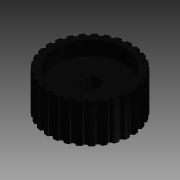
# Autodesk Inventor part: Llave hornillo
Saved by Autodesk Inventor 2014 (Build 180170000, 170)
## iProperties
Created: 2017-05-23
Part Number: Llave hornillo
Material: Generic
Document SubType Name: Modeling
Designer: resaj
Density: 1 g/cm^3
Appearance: Smooth - Black
Author: resaj
Autodesk Inventor part; units mm, degrees
ref_plane "YZ Plane" through (0, 0, 0) normal (1, 0, 0) x (0, 1, 0)
ref_plane "XZ Plane" through (0, 0, 0) normal (0, 1, 0) x (-1, 0, 0)
ref_plane "XY Plane" through (0, 0, 0) normal (0, 0, 1) x (1, 0, 0)
sketch "Sketch1" plane through (0, 0, 0) normal (0, 1, 0) x (-1, 0, 0)
  circle A0 centre (0, 0) radius 18.5
  dimension "d0" = 37
  constraints: 1 centre point, 1 coincident
  measures "d0" diameter of A0
extrude "Extrusion1" add sketch "Sketch1" along normal blind 17
sketch "Sketch2" plane through (0, 17, 0) normal (0, 1, 0) x (1, 0, 0)
  circle A0 centre (0, 0) radius 18.5 projected
  circle A1 centre (18.5, 0) radius 1
  line L0 (0, 0) -> (18.5, 0) construction
  dimension "d3" = 2
  constraints: 2 end point, 1 centre point, 1 horizontal, 1 horizontal alignment, 1 other
  measures "d3" diameter of A1
extrude "Extrusion2" cut sketch "Sketch2" against normal through all contours A0 A1 | A0 A1 picked at (18.1866, 0.2274) picked at (18.7982, 0.2581)
pattern_circular "Circular Pattern1" count 29 over 360 about axis through (0, 0, 0) along (0, 1, 0) of "Extrusion2"
sketch "Sketch3" plane through (0, 0, 0) normal (0, -1, 0) x (1, 0, 0)
  arc A0 (17.8262, 4.9474) -> (17.1854, 6.8494) centre (0, 0) ccw projected
hole "Hole1" at (0, 0, 0) direction (0, 1, 0) diameter 3.5 end through all countersink diameter 9.5 countersink angle 90
sketch "Sketch4" plane through (0, 0, 0) normal (0, -1, 0) x (1, 0, 0)
  circle A0 centre (0, 0) radius 4.75 projected
  arc A1 (-18.4728, 1.0035) -> (-18.4728, -1.0035) centre (0, 0) ccw projected
  arc A2 (18.473, 0.9996) -> (18.256, 2.9949) centre (0, 0) ccw projected
  line L0 (-9.6, 0.7) -> (-5.75, 0.7)
  line L1 (-5.75, 0.7) -> (-5.75, -0.7)
  line L2 (-5.75, -0.7) -> (-9.6, -0.7)
  line L3 (-9.6, -0.7) -> (-9.6, 0.7)
  line L4 (-18.5, 0) -> (0, 0) construction
  line L5 (-7.675, 0.7) -> (-7.675, 0) construction
  line L6 (-7.675, 0) -> (-7.675, -0.7) construction
  circle A3 centre (0, 0) radius 11.4692 construction
  line L7 (-0.2594, 7.791) -> (2.8062, 7.791) construction
  line L8 (2.8062, 7.791) -> (2.8062, 10.4034) construction
  line L9 (2.8062, 10.4034) -> (0.8969, 11.8689) construction
  line L10 (0.8969, 11.8689) -> (0.2634, 13.3204) construction
  line L11 (0.2634, 13.3204) -> (-0.0505, 15.6348) construction
  spline S0 degree 4 poles (-0.2594, 7.791) (2.8062, 7.791) (2.8062, 10.4034) (0.8969, 11.8689) (0.2634, 13.3204) (-0.0505, 15.6348) knots 1 1 1 1 1 2 3 3 3 3 3
  line L12 (-0.2594, 7.791) -> (-3.3031, 7.791) construction
  line L13 (-3.3031, 7.791) -> (-4.0256, 9.1624) construction
  line L14 (-4.0256, 9.1624) -> (-3.2524, 11.7471) construction
  spline S1 degree 3 poles (-0.2594, 7.791) (-3.3031, 7.791) (-4.0256, 9.1624) (-3.2524, 11.7471) knots 1 1 1 1 2 2 2 2
  line L15 (-3.2524, 11.7471) -> (-2.5295, 10.0909) construction
  line L16 (-2.5295, 10.0909) -> (-2.3206, 10.0909) construction
  line L17 (-2.3206, 10.0909) -> (-2.3206, 12.6773) construction
  line L18 (-2.3206, 12.6773) -> (-0.0505, 15.6348) construction
  spline S2 degree 4 poles (-3.2524, 11.7471) (-2.5295, 10.0909) (-2.3206, 10.0909) (-2.3206, 12.6773) (-0.0505, 15.6348) knots 1 1 1 1 1 2 2 2 2 2
  line L19 (5.6325, 5.7441) -> (6.9202, 4.4564) construction
  line L20 (6.9202, 4.4564) -> (8.0174, 5.5537) construction
  line L21 (8.0174, 5.5537) -> (7.8311, 6.9712) construction
  line L22 (7.8311, 6.9712) -> (8.1746, 7.8469) construction
  line L23 (8.1746, 7.8469) -> (9.0149, 8.9509) construction
  spline S3 degree 4 poles (5.6325, 5.7441) (6.9202, 4.4564) (8.0174, 5.5537) (7.8311, 6.9712) (8.1746, 7.8469) (9.0149, 8.9509) knots 1 1 1 1 1 2 3 3 3 3 3
  line L24 (5.6325, 5.7441) -> (4.354, 7.0226) construction
  line L25 (4.354, 7.0226) -> (4.6267, 7.9019) construction
  line L26 (4.6267, 7.9019) -> (6.0371, 8.6628) construction
  spline S4 degree 3 poles (5.6325, 5.7441) (4.354, 7.0226) (4.6267, 7.9019) (6.0371, 8.6628) knots 1 1 1 1 2 2 2 2
  line L27 (6.0371, 8.6628) -> (5.6451, 7.6636) construction
  line L28 (5.6451, 7.6636) -> (5.7328, 7.5758) construction
  line L29 (5.7328, 7.5758) -> (6.8191, 8.6622) construction
  line L30 (6.8191, 8.6622) -> (9.0149, 8.9509) construction
  spline S5 degree 4 poles (6.0371, 8.6628) (5.6451, 7.6636) (5.7328, 7.5758) (6.8191, 8.6622) (9.0149, 8.9509) knots 1 1 1 1 1 2 2 2 2 2
  arc A4 (18.256, -2.9949) -> (18.473, -0.9996) centre (0, 0) ccw projected
  line L31 (0, 0) -> (13.0815, 13.0815) construction
  line L32 (0, 0) -> (18.5, 0) construction
  spline S6 degree 2 poles (-10.161, -5.2239) (-10.0622, -5.4091) (-10.0419, -5.8018) (-10.129, -5.9928) knots 0 0 0 1 2 2 2
  spline S7 degree 2 poles (-10.129, -5.9928) (-10.2133, -6.1847) (-10.5824, -6.5424) (-10.8658, -6.6935) knots 0 0 0 1 2 2 2
  spline S8 degree 2 poles (-10.8658, -6.6935) (-11.1473, -6.8436) (-11.63, -6.9445) (-11.8463, -6.9106) knots 0 0 0 1 2 2 2
  spline S9 degree 2 poles (-11.8463, -6.9106) (-12.0571, -6.8783) (-12.3817, -6.6502) (-12.4843, -6.4576) knots 0 0 0 1 2 2 2
  spline S10 degree 2 poles (-12.4843, -6.4576) (-12.5356, -6.3614) (-12.592, -6.1768) (-12.6053, -6.0906) knots 0 0 0 1 2 2 2
  spline S11 degree 2 poles (-12.6053, -6.0906) (-12.6136, -6.0181) (-12.6161, -5.8515) (-12.6091, -5.7684) knots 0 0 0 1 2 2 2
  line L33 (-12.6091, -5.7684) -> (-12.2495, -5.5767)
  line L34 (-12.2495, -5.5767) -> (-12.2388, -5.5967)
  spline S12 degree 2 poles (-12.2388, -5.5967) (-12.2567, -5.6506) (-12.3033, -5.8083) (-12.3116, -5.9107) knots 0 0 0 1 2 2 2
  spline S13 degree 2 poles (-12.3116, -5.9107) (-12.3201, -6.0086) (-12.2891, -6.2113) (-12.229, -6.3239) knots 0 0 0 1 2 2 2
  spline S14 degree 2 poles (-12.229, -6.3239) (-12.1642, -6.4456) (-11.9309, -6.5988) (-11.7747, -6.6205) knots 0 0 0 1 2 2 2
  spline S15 degree 2 poles (-11.7747, -6.6205) (-11.6167, -6.6412) (-11.2223, -6.5453) (-11.0062, -6.4301) knots 0 0 0 1 2 2 2
  spline S16 degree 2 poles (-11.0062, -6.4301) (-10.7755, -6.3071) (-10.4934, -6.0355) (-10.4226, -5.8928) knots 0 0 0 1 2 2 2
  spline S17 degree 2 poles (-10.4226, -5.8928) (-10.3544, -5.7538) (-10.356, -5.4794) (-10.4199, -5.3595) knots 0 0 0 1 2 2 2
  spline S18 degree 2 poles (-10.4199, -5.3595) (-10.479, -5.2487) (-10.6413, -5.0973) (-10.7273, -5.0499) knots 0 0 0 1 2 2 2
  spline S19 degree 2 poles (-10.7273, -5.0499) (-10.8122, -5.0042) (-10.9645, -4.9548) (-11.0145, -4.9441) knots 0 0 0 1 2 2 2
  line L35 (-11.0145, -4.9441) -> (-11.0252, -4.9241)
  line L36 (-11.0252, -4.9241) -> (-10.6692, -4.7343)
  spline S20 degree 2 poles (-10.6692, -4.7343) (-10.6018, -4.7777) (-10.4781, -4.8564) (-10.4075, -4.919) knots 0 0 0 1 2 2 2
  spline S21 degree 2 poles (-10.4075, -4.919) (-10.3302, -4.9852) (-10.222, -5.1094) (-10.161, -5.2239) knots 0 0 0 1 2 2 2
  line L37 (-10.6086, -4.402) -> (-13.0032, -5.2488)
  line L38 (-13.0032, -5.2488) -> (-13.4534, -3.9757)
  line L39 (-13.4534, -3.9757) -> (-13.1701, -3.8755)
  line L40 (-13.1701, -3.8755) -> (-12.8153, -4.8788)
  line L41 (-12.8153, -4.8788) -> (-12.1594, -4.6469)
  line L42 (-12.1594, -4.6469) -> (-12.4901, -3.7115)
  line L43 (-12.4901, -3.7115) -> (-12.2068, -3.6113)
  line L44 (-12.2068, -3.6113) -> (-11.8761, -4.5467)
  line L45 (-11.8761, -4.5467) -> (-10.9873, -4.2324)
  line L46 (-10.9873, -4.2324) -> (-11.342, -3.2291)
  line L47 (-11.342, -3.2291) -> (-11.0587, -3.1289)
  line L48 (-11.0587, -3.1289) -> (-10.6086, -4.402)
  line L49 (-11.4486, -1.187) -> (-11.3791, -1.553)
  line L50 (-11.3791, -1.553) -> (-12.2447, -2.4128)
  line L51 (-12.2447, -2.4128) -> (-12.1837, -2.7343)
  line L52 (-12.1837, -2.7343) -> (-11.1908, -2.546)
  line L53 (-11.1908, -2.546) -> (-11.1374, -2.8271)
  line L54 (-11.1374, -2.8271) -> (-13.6329, -3.3005)
  line L55 (-13.6329, -3.3005) -> (-13.7365, -2.7544)
  spline S22 degree 2 poles (-13.7365, -2.7544) (-13.771, -2.5724) (-13.7713, -2.3169) (-13.7075, -2.1895) knots 0 0 0 1 2 2 2
  spline S23 degree 2 poles (-13.7075, -2.1895) (-13.6437, -2.0622) (-13.4033, -1.8825) (-13.2071, -1.8453) knots 0 0 0 1 2 2 2
  spline S24 degree 2 poles (-13.2071, -1.8453) (-12.9341, -1.7935) (-12.5192, -1.9599) (-12.3914, -2.1473) knots 0 0 0 1 2 2 2
  line L56 (-12.3914, -2.1473) -> (-11.4486, -1.187)
  spline S25 degree 2 poles (-13.1252, -2.1336) (-13.2344, -2.1543) (-13.39, -2.2508) (-13.4316, -2.33) knots 0 0 0 1 2 2 2
  spline S26 degree 2 poles (-13.4316, -2.33) (-13.4666, -2.3994) (-13.4747, -2.5665) (-13.452, -2.6858) knots 0 0 0 1 2 2 2
  line L57 (-13.452, -2.6858) -> (-13.3991, -2.9649)
  line L58 (-13.3991, -2.9649) -> (-12.4608, -2.7869)
  line L59 (-12.4608, -2.7869) -> (-12.5079, -2.5381)
  spline S27 degree 2 poles (-12.5079, -2.5381) (-12.531, -2.4168) (-12.6183, -2.2323) (-12.7103, -2.1785) knots 0 0 0 1 2 2 2
  spline S28 degree 2 poles (-12.7103, -2.1785) (-12.7905, -2.1308) (-12.9958, -2.109) (-13.1252, -2.1336) knots 0 0 0 1 2 2 2
  line L60 (-11.4914, 0.6533) -> (-11.4812, 0.2809)
  line L61 (-11.4812, 0.2809) -> (-12.4728, -0.4299)
  line L62 (-12.4728, -0.4299) -> (-12.4638, -0.7571)
  line L63 (-12.4638, -0.7571) -> (-11.4535, -0.7294)
  line L64 (-11.4535, -0.7294) -> (-11.4457, -1.0154)
  line L65 (-11.4457, -1.0154) -> (-13.9848, -1.0849)
  line L66 (-13.9848, -1.0849) -> (-14, -0.5294)
  spline S29 degree 2 poles (-14, -0.5294) (-14.005, -0.3442) (-13.9646, -0.0919) (-13.8812, 0.0237) knots 0 0 0 1 2 2 2
  spline S30 degree 2 poles (-13.8812, 0.0237) (-13.7979, 0.1392) (-13.532, 0.2783) (-13.3324, 0.2837) knots 0 0 0 1 2 2 2
  spline S31 degree 2 poles (-13.3324, 0.2837) (-13.0546, 0.2913) (-12.6715, 0.0609) (-12.5753, -0.1444) knots 0 0 0 1 2 2 2
  line L67 (-12.5753, -0.1444) -> (-11.4914, 0.6533)
  spline S32 degree 2 poles (-13.2975, -0.0139) (-13.4086, -0.0169) (-13.5776, -0.0874) (-13.6312, -0.1589) knots 0 0 0 1 2 2 2
  spline S33 degree 2 poles (-13.6312, -0.1589) (-13.6769, -0.2219) (-13.7115, -0.3856) (-13.7082, -0.507) knots 0 0 0 1 2 2 2
  line L68 (-13.7082, -0.507) -> (-13.7004, -0.7909)
  line L69 (-13.7004, -0.7909) -> (-12.7457, -0.7648)
  line L70 (-12.7457, -0.7648) -> (-12.7526, -0.5117)
  spline S34 degree 2 poles (-12.7526, -0.5117) (-12.756, -0.3882) (-12.8128, -0.1921) (-12.895, -0.1244) knots 0 0 0 1 2 2 2
  spline S35 degree 2 poles (-12.895, -0.1244) (-12.9666, -0.0645) (-13.1658, -0.0103) (-13.2975, -0.0139) knots 0 0 0 1 2 2 2
  line L71 (-11.4907, 0.5916) -> (-13.9137, 1.6445)
  line L72 (-13.9137, 1.6445) -> (-13.8673, 1.9955)
  line L73 (-13.8673, 1.9955) -> (-11.254, 2.3833)
  line L74 (-11.254, 2.3833) -> (-11.2936, 2.0833)
  line L75 (-11.2936, 2.0833) -> (-12.0233, 1.9824)
  line L76 (-12.0233, 1.9824) -> (-12.1313, 1.1641)
  line L77 (-12.1313, 1.1641) -> (-11.4529, 0.8773)
  line L78 (-11.4529, 0.8773) -> (-11.4907, 0.5916)
  line L79 (-12.3192, 1.9426) -> (-13.5525, 1.7692)
  line L80 (-13.5525, 1.7692) -> (-12.4065, 1.2814)
  line L81 (-12.4065, 1.2814) -> (-12.3192, 1.9426)
  spline S36 degree 2 poles (-11.9106, 4.605) (-11.578, 4.5031) (-11.1127, 4.1108) (-11.0222, 3.8721) knots 0 0 0 1 2 2 2
  spline S37 degree 2 poles (-11.0222, 3.8721) (-10.9537, 3.681) (-10.9739, 3.3341) (-11.0511, 3.0822) knots 0 0 0 1 2 2 2
  line L82 (-11.0511, 3.0822) -> (-11.1965, 2.6079)
  line L83 (-11.1965, 2.6079) -> (-13.625, 3.3522)
  line L84 (-13.625, 3.3522) -> (-13.4808, 3.8225)
  spline S38 degree 2 poles (-13.4808, 3.8225) (-13.3922, 4.1118) (-13.1885, 4.4111) (-13.0618, 4.5014) knots 0 0 0 1 2 2 2
  spline S39 degree 2 poles (-13.0618, 4.5014) (-12.8454, 4.6526) (-12.2648, 4.7136) (-11.9106, 4.605) knots 0 0 0 1 2 2 2
  spline S40 degree 2 poles (-12.002, 4.3209) (-12.2814, 4.4065) (-12.7252, 4.3703) (-12.8851, 4.2492) knots 0 0 0 1 2 2 2
  spline S41 degree 2 poles (-12.8851, 4.2492) (-12.9956, 4.1625) (-13.1405, 3.9357) (-13.1978, 3.7487) knots 0 0 0 1 2 2 2
  line L85 (-13.1978, 3.7487) -> (-13.2617, 3.5401)
  line L86 (-13.2617, 3.5401) -> (-11.3921, 2.9671)
  line L87 (-11.3921, 2.9671) -> (-11.3282, 3.1757)
  spline S42 degree 2 poles (-11.3282, 3.1757) (-11.2721, 3.3588) (-11.2565, 3.6554) (-11.3146, 3.7959) knots 0 0 0 1 2 2 2
  spline S43 degree 2 poles (-11.3146, 3.7959) (-11.3847, 3.9746) (-11.7186, 4.234) (-12.002, 4.3209) knots 0 0 0 1 2 2 2
  spline S44 degree 2 poles (-11.8745, 6.9059) (-11.6679, 6.9383) (-11.1666, 6.8327) (-10.8848, 6.6874) knots 0 0 0 1 2 2 2
  spline S45 degree 2 poles (-10.8848, 6.6874) (-10.6104, 6.5459) (-10.2272, 6.1978) (-10.1347, 6.0089) knots 0 0 0 1 2 2 2
  spline S46 degree 2 poles (-10.1347, 6.0089) (-10.0377, 5.8107) (-10.049, 5.4205) (-10.1461, 5.232) knots 0 0 0 1 2 2 2
  spline S47 degree 2 poles (-10.1461, 5.232) (-10.247, 5.0363) (-10.5629, 4.8054) (-10.7732, 4.7703) knots 0 0 0 1 2 2 2
  spline S48 degree 2 poles (-10.7732, 4.7703) (-10.9798, 4.7379) (-11.4821, 4.8463) (-11.7601, 4.9896) knots 0 0 0 1 2 2 2
  spline S49 degree 2 poles (-11.7601, 4.9896) (-12.0437, 5.1358) (-12.4132, 5.4792) (-12.5122, 5.6691) knots 0 0 0 1 2 2 2
  spline S50 degree 2 poles (-12.5122, 5.6691) (-12.6046, 5.8581) (-12.5989, 6.2511) (-12.4989, 6.445) knots 0 0 0 1 2 2 2
  spline S51 degree 2 poles (-12.4989, 6.445) (-12.3979, 6.6408) (-12.0747, 6.8724) (-11.8745, 6.9059) knots 0 0 0 1 2 2 2
  spline S52 degree 2 poles (-11.0216, 6.4221) (-11.2448, 6.5372) (-11.633, 6.6331) (-11.7851, 6.6166) knots 0 0 0 1 2 2 2
  spline S53 degree 2 poles (-11.7851, 6.6166) (-11.9418, 6.6001) (-12.1693, 6.4465) (-12.2391, 6.3111) knots 0 0 0 1 2 2 2
  spline S54 degree 2 poles (-12.2391, 6.3111) (-12.3108, 6.172) (-12.3039, 5.9068) (-12.2247, 5.7641) knots 0 0 0 1 2 2 2
  spline S55 degree 2 poles (-12.2247, 5.7641) (-12.149, 5.6278) (-11.8429, 5.3681) (-11.6234, 5.2549) knots 0 0 0 1 2 2 2
  spline S56 degree 2 poles (-11.6234, 5.2549) (-11.1788, 5.0257) (-10.5436, 5.0989) (-10.4059, 5.366) knots 0 0 0 1 2 2 2
  spline S57 degree 2 poles (-10.4059, 5.366) (-10.2682, 5.6331) (-10.577, 6.1929) (-11.0216, 6.4221) knots 0 0 0 1 2 2 2
  dimension "d16" = 1.4
  dimension "d17" = 3.85
  dimension "d18" = 1
  dimension "d21" = 0.7224
  dimension "d23" = 2.5841
  dimension "d24" = 0.6335
  dimension "d25" = 1.9093
  dimension "d26" = 1.3714
  dimension "d27" = 0.9285
  dimension "d28" = 0.3125
  dimension "d30" = 0.8084
  dimension "d31" = 0.6431
  dimension "d32" = 2.3144
  dimension "d33" = 1.3437
  dimension "d34" = 0.1218
  dimension "d48" = 0.0508
  dimension "d50" = 0.2089
  dimension "d81" = 45
  constraints: 18 end point, 8 parallel, 5 perpendicular, 2 equal length, 2 horizontal, 2 midpoint, 2 point on circle, 1 centre point, 1 coincident, 1 point on line, 1 vertical, 19 other
  measures "d16" distance of L0.end L1.end
  measures "d17" distance of L0.start L0.end
  measures "d18" distance edge to line of A0 L1
  measures "d21" horizontal distance of L12.end L13.end
  measures "d23" horizontal distance of L10.end L16.end
  measures "d24" horizontal distance of L9.end L10.end
  measures "d25" horizontal distance of L7.end L9.end
  measures "d26" vertical distance of L13.end L12.end
  measures "d27" vertical distance of L16.end L13.end
  measures "d28" vertical distance of L8.end L16.end
  measures "d30" vertical distance of L17.end L9.end
  measures "d31" vertical distance of L10.end L17.end
  measures "d32" vertical distance of L11.end L10.end
  measures "d33" vertical distance of L14.end L8.end
  measures "d34" vertical distance of L9.end L14.end
  measures "d48" horizontal distance of L14.end L12.end
  measures "d50" distance of L15.end L16.end
  measures "d81" angle of L32 L31
extrude "Extrusion3" cut sketch "Sketch4" against normal blind 1 contours L0 L1 L2 L3 | S1 S2 S0 | S4 S5 S3 | S6 S7 S8 S9 S10 S11 L33 L34 S12 S13 S14 S15 S16 S17 S18 S19 L35 L36 S20 S21 | L37 L38 L39 L40 L41 L42 L43 L44 L45 L46 L47 L48 | L49 L50 L51 L52 L53 L54 L55 S22 S23 S24 L56 | L67 L71 L72 L73 L74 L75 L76 L77 L78 L60 | L60 L71 L67 | L60 L61 L62 L63 L64 L65 L66 S29 S30 S31 L67 L71 | S36 S37 L82 L83 L84 S38 S39 | S44 S45 S46 S47 S48 S49 S50 S51
sketch "Sketch5" plane through (0, 17, 0) normal (0, 1, 0) x (1, 0, 0)
  circle A0 centre (0, 0) radius 1.75 projected
  arc A1 (17.1854, -6.8494) -> (17.8262, -4.9474) centre (0, 0) ccw projected
  circle A2 centre (0, 0) radius 15.15
  dimension "d82" = 30.3
  constraints: 1 centre point, 1 coincident
  measures "d82" diameter of A2
extrude "Extrusion4" cut sketch "Sketch5" against normal blind 6.25
sketch "Sketch6" plane through (0, 10.75, 0) normal (0, 1, 0) x (1, 0, 0)
  circle A0 centre (0, 0) radius 1.75 projected
  circle A1 centre (0, 0) radius 15.15 projected
  circle A2 centre (0, 0) radius 4.2
  line L0 (-2.5001, 3.3748) -> (-2.6767, 1.7494)
  line L1 (3.1666, 2.7592) -> (2.9899, 1.1337)
  line L2 (-2.5001, 3.3748) -> (3.1666, 2.7592) construction
  line L3 (-2.6767, 1.7494) -> (-2.9749, 1.7818)
  line L4 (-2.9749, 1.7818) -> (-3.2882, -1.1013)
  line L5 (-3.2882, -1.1013) -> (-2.9899, -1.1337)
  line L6 (-2.9899, -1.1337) -> (2.6767, -1.7494) construction
  line L7 (-2.6767, 1.7494) -> (2.9899, 1.1337) construction
  line L8 (2.9899, 1.1337) -> (3.2882, 1.1013)
  line L9 (3.2882, 1.1013) -> (2.9749, -1.7818)
  line L10 (2.9749, -1.7818) -> (2.6767, -1.7494)
  line L11 (-3.1316, 0.3402) -> (0, 0) construction
  line L12 (-2.9899, -1.1337) -> (-3.1666, -2.7592)
  line L13 (-2.6767, 1.7494) -> (-2.9899, -1.1337) construction
  line L14 (2.9899, 1.1337) -> (2.6767, -1.7494) construction
  line L15 (2.6767, -1.7494) -> (2.5001, -3.3748)
  circle A3 centre (0, 0) radius 15.15 construction
  arc A4 (18.256, -2.9949) -> (17.8262, -4.9474) centre (18.0675, -3.977) ccw construction
  arc A5 (18.256, -2.9949) -> (18.473, -0.9996) centre (0, 0) ccw construction
  arc A6 (18.473, 0.9996) -> (18.473, -0.9996) centre (18.5, 0) ccw construction
  arc A7 (18.473, 0.9996) -> (18.256, 2.9949) centre (0, 0) ccw construction
  arc A8 (17.8262, 4.9474) -> (18.256, 2.9949) centre (18.0675, 3.977) ccw construction
  arc A9 (17.8262, 4.9474) -> (17.1854, 6.8494) centre (0, 0) ccw construction
  arc A10 (16.3459, 8.6638) -> (17.1854, 6.8494) centre (16.7901, 7.7679) ccw construction
  arc A11 (16.3459, 8.6638) -> (15.3112, 10.3836) centre (0, 0) ccw construction
  arc A12 (14.1013, 11.9752) -> (15.3112, 10.3836) centre (14.7277, 11.1957) ccw construction
  arc A13 (14.1013, 11.9752) -> (12.721, 13.4322) centre (0, 0) ccw construction
  arc A14 (11.1973, 14.7265) -> (12.721, 13.4322) centre (11.9766, 14.1) ccw construction
  arc A15 (11.1973, 14.7265) -> (9.5361, 15.8529) centre (0, 0) ccw construction
  arc A16 (7.7697, 16.7893) -> (9.5361, 15.8529) centre (8.6656, 16.345) ccw construction
  arc A17 (7.7697, 16.7893) -> (5.9052, 17.5322) centre (0, 0) ccw construction
  arc A18 (3.9788, 18.0671) -> (5.9052, 17.5322) centre (4.9493, 17.8257) ccw construction
  arc A19 (3.9788, 18.0671) -> (1.9983, 18.3918) centre (0, 0) ccw construction
  arc A20 (0.0019, 18.5) -> (1.9983, 18.3918) centre (1.0016, 18.4729) ccw construction
  arc A21 (0.0019, 18.5) -> (-2.0021, 18.3913) centre (0, 0) ccw construction
  arc A22 (-3.9751, 18.0679) -> (-2.0021, 18.3913) centre (-2.993, 18.2563) ccw construction
  arc A23 (-3.9751, 18.0679) -> (-5.9089, 17.531) centre (0, 0) ccw construction
  arc A24 (-7.7662, 16.791) -> (-5.9089, 17.531) centre (-6.8476, 17.1861) ccw construction
  arc A25 (-7.7662, 16.791) -> (-9.5394, 15.8509) centre (0, 0) ccw construction
  arc A26 (-11.1942, 14.7289) -> (-9.5394, 15.8509) centre (-10.382, 15.3122) ccw construction
  arc A27 (-11.1942, 14.7289) -> (-12.7238, 13.4296) centre (0, 0) ccw construction
  arc A28 (-14.0987, 11.9781) -> (-12.7238, 13.4296) centre (-13.4309, 12.7224) ccw construction
  arc A29 (-14.0987, 11.9781) -> (-15.3133, 10.3804) centre (0, 0) ccw construction
  arc A30 (-16.3441, 8.6673) -> (-15.3133, 10.3804) centre (-15.8519, 9.5377) ccw construction
  arc A31 (-16.3441, 8.6673) -> (-17.1868, 6.8458) centre (0, 0) ccw construction
  arc A32 (-17.8252, 4.9511) -> (-17.1868, 6.8458) centre (-17.5316, 5.9071) ccw construction
  arc A33 (-17.8252, 4.9511) -> (-18.2566, 2.9911) centre (0, 0) ccw construction
  arc A34 (-18.4728, 1.0035) -> (-18.2566, 2.9911) centre (-18.3916, 2.0002) ccw construction
  arc A35 (-18.4728, 1.0035) -> (-18.4728, -1.0035) centre (0, 0) ccw construction
  arc A36 (-18.2566, -2.9911) -> (-18.4728, -1.0035) centre (-18.3916, -2.0002) ccw construction
  arc A37 (-18.2566, -2.9911) -> (-17.8252, -4.9511) centre (0, 0) ccw construction
  arc A38 (-17.1868, -6.8458) -> (-17.8252, -4.9511) centre (-17.5316, -5.9071) ccw construction
  arc A39 (-17.1868, -6.8458) -> (-16.3441, -8.6673) centre (0, 0) ccw construction
  arc A40 (-15.3133, -10.3804) -> (-16.3441, -8.6673) centre (-15.8519, -9.5377) ccw construction
  arc A41 (-15.3133, -10.3804) -> (-14.0987, -11.9781) centre (0, 0) ccw construction
  arc A42 (-12.7238, -13.4296) -> (-14.0987, -11.9781) centre (-13.4309, -12.7224) ccw construction
  arc A43 (-12.7238, -13.4296) -> (-11.1942, -14.7289) centre (0, 0) ccw construction
  arc A44 (-9.5394, -15.8509) -> (-11.1942, -14.7289) centre (-10.382, -15.3122) ccw construction
  arc A45 (-9.5394, -15.8509) -> (-7.7662, -16.791) centre (0, 0) ccw construction
  arc A46 (-5.9089, -17.531) -> (-7.7662, -16.791) centre (-6.8476, -17.1861) ccw construction
  arc A47 (-5.9089, -17.531) -> (-3.9751, -18.0679) centre (0, 0) ccw construction
  arc A48 (-2.0021, -18.3913) -> (-3.9751, -18.0679) centre (-2.993, -18.2563) ccw construction
  arc A49 (-2.0021, -18.3913) -> (0.0019, -18.5) centre (0, 0) ccw construction
  arc A50 (1.9983, -18.3918) -> (0.0019, -18.5) centre (1.0016, -18.4729) ccw construction
  arc A51 (1.9983, -18.3918) -> (3.9788, -18.0671) centre (0, 0) ccw construction
  arc A52 (5.9052, -17.5322) -> (3.9788, -18.0671) centre (4.9493, -17.8257) ccw construction
  arc A53 (5.9052, -17.5322) -> (7.7697, -16.7893) centre (0, 0) ccw construction
  arc A54 (9.5361, -15.8529) -> (7.7697, -16.7893) centre (8.6656, -16.345) ccw construction
  arc A55 (9.5361, -15.8529) -> (11.1973, -14.7265) centre (0, 0) ccw construction
  arc A56 (12.721, -13.4322) -> (11.1973, -14.7265) centre (11.9766, -14.1) ccw construction
  arc A57 (12.721, -13.4322) -> (14.1013, -11.9752) centre (0, 0) ccw construction
  arc A58 (15.3112, -10.3836) -> (14.1013, -11.9752) centre (14.7277, -11.1957) ccw construction
  arc A59 (15.3112, -10.3836) -> (16.3459, -8.6638) centre (0, 0) ccw construction
  arc A60 (17.1854, -6.8494) -> (16.3459, -8.6638) centre (16.7901, -7.7679) ccw construction
  arc A61 (17.1854, -6.8494) -> (17.8262, -4.9474) centre (0, 0) ccw construction
  line L16 (1.9983, 18.3918) -> (0, 0) construction
  dimension "d85" = 8.4
  dimension "d86" = 5.7
  dimension "d87" = 2.9
  dimension "d88" = 6.3
  constraints: 34 end point, 18 parallel, 15 perpendicular, 4 point on circle, 2 collinear, 1 centre point, 1 coincident, 1 midpoint, 1 point on line
  measures "d85" diameter of A2
  measures "d86" distance between parallel lines of L1 L0
  measures "d87" distance of L3.end L4.end
  measures "d88" distance between parallel lines of L9 L4
extrude "Extrusion5" cut sketch "Sketch6" against normal blind 5.5 contours L1 L8 L9 L10 L15 A2 L12 L5 L4 L3 L0
body "Solid1"
